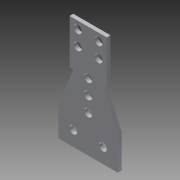
# Autodesk Inventor part: that thing mount
Saved by Autodesk Inventor 2013 (Build 170138000, 138)
## iProperties
Created: 2013-02-04
Part Number: that thing mount
Material: Aluminum 6061
Document SubType Name: Modeling
Designer: Arpan
Density: 1 g/cm^3
Author: Arpan
Autodesk Inventor part; units mm, degrees
ref_plane "YZ Plane" through (0, 0, 0) normal (1, 0, 0) x (0, 1, 0)
ref_plane "XZ Plane" through (0, 0, 0) normal (0, 1, 0) x (-1, 0, 0)
ref_plane "XY Plane" through (0, 0, 0) normal (0, 0, 1) x (1, 0, 0)
sketch "Sketch1" plane through (0, 0, 0) normal (0, 0, 1) x (1, 0, 0)
  line L0 (0, 0) -> (-50.8, 0)
  line L1 (-50.8, 0) -> (-50.8, 57.15)
  line L2 (-50.8, 57.15) -> (0, 57.15)
  line L3 (0, 57.15) -> (0, 0)
  line L4 (-50.8, 0) -> (-50.8, 25.4)
  line L5 (0, 0) -> (0, 25.4)
  line L6 (-25.4, 57.15) -> (-38.1, 57.15)
  line L7 (-25.4, 57.15) -> (-12.7, 57.15)
  line L8 (-12.7, 57.15) -> (0, 28.575)
  line L9 (-38.1, 57.15) -> (-50.8, 25.4)
  dimension "d0" = 50.8
  dimension "d1" = 57.15
  dimension "d2" = 25.4
  dimension "d3" = 12.7
  dimension "d4" = 12.7
  constraints: 20 end point, 4 point on line, 2 midpoint, 2 parallel, 1 horizontal, 1 perpendicular
  measures "d0" distance of L0.start L0.end
  measures "d1" distance of L0.end L1.end
  measures "d2" distance of L0.end L4.end
  measures "d3" distance of L6.start L6.end
  measures "d4" distance of L6.start L7.end
extrude "Extrusion1" add sketch "Sketch1" along normal blind 3.175 contours L0 L1 L9 L2 L8 L3
sketch "Sketch2" plane through (0, 0, 3.175) normal (0, 0, 1) x (1, 0, 0)
  line L0 (-12.7, 57.15) -> (-38.1, 57.15) projected
  line L1 (-50.8, 0) -> (0, 0) projected
  line L2 (-38.1, 57.15) -> (-38.1, 95.25)
  line L3 (-38.1, 95.25) -> (-12.7, 95.25)
  line L4 (-12.7, 95.25) -> (-12.7, 57.15)
  dimension "d7" = 38.1
  constraints: 6 end point, 2 perpendicular, 1 parallel
  measures "d7" distance of L0.end L2.end
extrude "Extrusion2" add sketch "Sketch2" against normal blind 3.175
sketch "Sketch3" plane through (0, 0, 0) normal (0, 0, -1) x (-1, 0, 0)
  circle A0 centre (25.4, 57.15) radius 3.3782 projected
  circle A1 centre (25.4, 44.45) radius 3.3782 projected
  circle A2 centre (25.4, 31.75) radius 3.3782 projected
  circle A3 centre (12.7, 12.7) radius 3.302 projected
  circle A4 centre (38.1, 12.7) radius 3.302 projected
extrude "Extrusion3" cut sketch "Sketch3" against normal blind 3.175
sketch "Sketch4" plane through (0, 0, 3.175) normal (0, 0, 1) x (1, 0, 0)
  line L0 (-12.7, 95.25) -> (-38.1, 95.25) projected
  line L1 (-38.1, 95.25) -> (-34.29, 95.25)
  line L2 (-34.29, 95.25) -> (-34.29, 88.9)
  line L3 (-34.29, 88.9) -> (-34.29, 76.2)
  line L4 (-12.7, 95.25) -> (-16.51, 95.25)
  line L5 (-16.51, 95.25) -> (-16.51, 88.9)
  line L6 (-16.51, 88.9) -> (-16.51, 82.55)
  circle A0 centre (-34.29, 88.9) radius 3.3782
  circle A1 centre (-16.51, 88.9) radius 3.3782
  circle A2 centre (-34.29, 76.2) radius 3.3782
  line L7 (-16.51, 88.9) -> (-16.51, 76.2)
  circle A3 centre (-16.51, 76.2) radius 3.3782
  dimension "d12" = 3.81
  dimension "d13" = 6.35
  dimension "d14" = 12.7
  dimension "d15" = 3.81
  dimension "d16" = 6.7564
  dimension "d17" = 6.7564
  dimension "d18" = 6.7564
  dimension "d19" = 6.7564
  constraints: 14 end point, 4 centre point, 4 coincident, 3 perpendicular, 3 point on line, 1 collinear
  measures "d12" distance of L0.end L1.end
  measures "d13" distance of L1.end L2.end
  measures "d14" distance of L2.end L3.end
  measures "d15" distance of L0.start L4.end
  measures "d16" diameter of A0
  measures "d17" diameter of A1
  measures "d18" diameter of A2
  measures "d19" diameter of A3
extrude "Extrusion4" cut sketch "Sketch4" against normal blind 25.4
sketch "Sketch5" plane through (-12.7, 57.15, 3.175) normal (1, 0, 0) x (0, 0, -1)
  line L0 (0, 0) -> (0, 38.1) projected
  line L1 (3.175, 0) -> (0, 0) projected
  line L2 (3.175, 38.1) -> (3.175, 0) projected
  line L3 (0, 38.1) -> (3.175, 38.1) projected
  point P0 (3.175, -57.15)
extrude "Extrusion5" add sketch "Sketch5" along normal blind 3.175
sketch "Sketch6" plane through (-38.1, 57.15, 3.175) normal (-1, 0, 0) x (0, 0, 1)
  line L0 (0, 38.1) -> (0, 0) projected
  line L1 (0, 38.1) -> (-3.175, 38.1) projected
  line L2 (-3.175, 0) -> (-3.175, 38.1) projected
  line L3 (-3.175, 0) -> (0, 0) projected
  point P0 (-3.175, -57.15)
extrude "Extrusion6" add sketch "Sketch6" along normal blind 3.175
body "Solid1"
